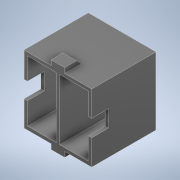
# Autodesk Inventor part: caixaled_pt1
Saved by Autodesk Inventor 2022 (Build 260153000, 153)
## iProperties
Created: 2024-02-25
Part Number: caixaled_pt1
Material: Plástico PC/ABS
Document SubType Name: Modeling
Designer: Daniel
Density: 0.357273 g/cm^3
Appearance: Suave - Preto
Author: Daniel
Autodesk Inventor part; units mm, degrees
ref_plane "YZ Plane" through (0, 0, 0) normal (1, 0, 0) x (0, 1, 0)
ref_plane "XZ Plane" through (0, 0, 0) normal (0, 1, 0) x (-1, 0, 0)
ref_plane "XY Plane" through (0, 0, 0) normal (0, 0, 1) x (1, 0, 0)
sketch "Esboço1" plane through (0, 0, 0) normal (0, 0, 1) x (1, 0, 0)
  line L0 (0, 0) -> (20, 0)
  line L1 (20, 0) -> (20, 20)
  line L2 (20, 20) -> (0, 20)
  line L3 (0, 20) -> (0, 0)
  dimension "d0" = 20
  dimension "d1" = 20
  constraints: 8 end point, 2 parallel, 1 horizontal, 1 perpendicular
  measures "d0" distance of L2.end L1.end
  measures "d1" distance of L1.end L0.end
extrude "Extrusão1" add sketch "Esboço1" along normal blind 1
sketch "Esboço2" plane through (0, 0, 1) normal (0, 0, 1) x (1, 0, 0)
  circle A0 centre (7.25, 10) radius 1.5
  circle A1 centre (12.75, 10) radius 1.5
  line L0 (0, 0) -> (20, 0) projected
  line L1 (20, 0) -> (20, 20) projected
  dimension "d4" = 3
  dimension "d5" = 3
  dimension "d6" = 5.5
  dimension "d7" = 10
  dimension "d8" = 10
  dimension "d9" = 7.25
  constraints: 2 centre point
  measures "d4" diameter of A1
  measures "d5" diameter of A0
  measures "d6" distance of A1.centre A0.centre
  measures "d7" distance from line of L0 A1.centre
  measures "d8" distance from line of L0 A0.centre
  measures "d9" distance from line of L1 A1.centre
extrude "Extrusão2" cut sketch "Esboço2" against normal blind 1
sketch "Esboço3" plane through (0, 0, 1) normal (0, 0, 1) x (1, 0, 0)
  circle A0 centre (7.25, 10) radius 1.5 projected
  circle A1 centre (7.25, 10) radius 2
  circle A2 centre (12.75, 10) radius 1.5 projected
  circle A3 centre (12.75, 10) radius 2
  point P0 (0, 0)
  dimension "d12" = 4
  dimension "d13" = 4
  constraints: 2 centre point, 2 coincident
  measures "d12" diameter of A1
  measures "d13" diameter of A3
extrude "Extrusão3" add sketch "Esboço3" along normal blind 5
sketch "Esboço4" plane through (0, 0, 1) normal (0, 0, 1) x (1, 0, 0)
  line L0 (20, 20) -> (0, 20) projected
  line L1 (10.5, 20) -> (9.5, 20)
  line L2 (9.5, 20) -> (9.5, 0)
  line L3 (9.5, 0) -> (10.5, 0)
  line L4 (10.5, 0) -> (10.5, 20)
  line L5 (0, 20) -> (0, 0) projected
  line L6 (20, 0) -> (20, 20) projected
  line L7 (0, 0) -> (20, 0) projected
  line L8 (1, 19) -> (19, 19)
  line L9 (19, 19) -> (19, 1)
  line L10 (19, 1) -> (1, 1)
  line L11 (1, 1) -> (1, 19)
  point P0 (9.5, 0)
  point P1 (10.5, 19)
  point P2 (10.5, 1)
  point P3 (9.5, 19)
  point P4 (9.5, 1)
  dimension "d16" = 9.5
  dimension "d17" = 9.5
  dimension "d18" = 0
  dimension "d19" = 1
  constraints: 16 end point, 2 parallel, 1 horizontal, 1 perpendicular, 1 point on line, 3 other
  measures "d16" distance between parallel lines of L5 L2
  measures "d17" distance between parallel lines of L6 L4
  measures "d18" distance between parallel lines of L7 L3
  measures "d19" distance between parallel lines of L0 L8
extrude "Extrusão4" add sketch "Esboço4" along normal blind 18 contours L6 L7 L4 L10 L9 L8 L0 | L4 L8 L2 L0 | L2 L8 L11 L10 L7 L5 L0 | L4 L10 L2 L8 | L3 L2 L10 L4
sketch "Esboço5" plane through (0, 0, 19) normal (0, 0, 1) x (1, 0, 0)
  line L0 (0, 20) -> (0, 0) projected
  line L1 (1, 1) -> (1, 19) projected
  line L2 (0, 7.5) -> (1, 7.5)
  line L3 (1, 7.5) -> (1, 12.5)
  line L4 (1, 12.5) -> (0, 12.5)
  line L5 (0, 12.5) -> (0, 7.5)
  line L6 (19, 1) -> (19, 19) projected
  line L7 (20, 0) -> (20, 20) projected
  line L8 (19, 7.5) -> (20, 7.5)
  line L9 (20, 7.5) -> (20, 12.5)
  line L10 (20, 12.5) -> (19, 12.5)
  line L11 (19, 12.5) -> (19, 7.5)
  line L12 (20, 20) -> (0, 20) projected
  point P0 (0, 12.5)
  dimension "d22" = 5
  dimension "d23" = 7.5
  dimension "d24" = 5
  dimension "d25" = 7.5
  constraints: 16 end point, 4 parallel, 4 point on line, 2 horizontal, 2 perpendicular
  measures "d22" distance between parallel lines of L10 L8
  measures "d23" distance between parallel lines of L12 L10
  measures "d24" distance between parallel lines of L2 L4
  measures "d25" distance between parallel lines of L12 L4
extrude "Extrusão5" cut sketch "Esboço5" against normal blind 5
sketch "Esboço6" plane through (0, 0, 19) normal (0, 0, 1) x (1, 0, 0)
  line L0 (20, 20) -> (0, 20) projected
  line L1 (8, 20) -> (12, 20)
  line L2 (12, 20) -> (12, 21.5)
  line L3 (12, 21.5) -> (8, 21.5)
  line L4 (8, 21.5) -> (8, 20)
  line L5 (0, 0) -> (20, 0) projected
  line L6 (12, 0) -> (8, 0)
  line L7 (8, 0) -> (8, -1.5)
  line L8 (8, -1.5) -> (12, -1.5)
  line L9 (12, -1.5) -> (12, 0)
  dimension "d28" = 8
  dimension "d29" = 8
  dimension "d30" = 1.5
  dimension "d36" = 1.5
  dimension "d37" = 8
  dimension "d38" = 8
  constraints: 16 end point, 4 parallel, 2 horizontal, 2 perpendicular, 2 point on line
  measures "d28" distance from line of L0.start L2
  measures "d29" distance from line of L0.end L4
  measures "d30" distance of L3.end L1.start
  measures "d36" distance of L8.end L6.start
  measures "d37" distance from line of L5.start L7
  measures "d38" distance from line of L5.end L9
extrude "Extrusão6" add sketch "Esboço6" against normal blind 5
chamfer "Chanfro1" distance 1.5 angle 45 2 edges at (10, 21.5, 14) (10, -1.5, 14)
